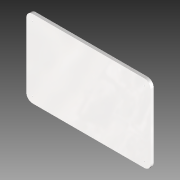
# Autodesk Inventor part: 4103_Aluminum Box Bottom_V1
Saved by Autodesk Inventor 2020 (Build 240168000, 168)
## iProperties
Created: 2020-09-13
Part Number: 4103_Aluminum Box Bottom_V1
Material: UHMW, White
Document SubType Name: Modeling
Designer: Eli Mattingly
Density: 0.94 g/cm^3
Appearance: Smooth - White
Author: Eli Mattingly
Autodesk Inventor part; units mm, degrees
ref_plane "YZ Plane" through (0, 0, 0) normal (1, 0, 0) x (0, 1, 0)
ref_plane "XZ Plane" through (0, 0, 0) normal (0, 1, 0) x (-1, 0, 0)
ref_plane "XY Plane" through (0, 0, 0) normal (0, 0, 1) x (1, 0, 0)
sketch "Sketch1" plane through (0, 0, 0) normal (0, 0, 1) x (1, 0, 0)
  line L0 (-200, 125) -> (200, 125)
  line L1 (200, 125) -> (200, -125)
  line L2 (200, -125) -> (-200, -125)
  line L3 (-200, -125) -> (-200, 125)
  line L4 (-200, 125) -> (200, -125) construction
  line L5 (200, 125) -> (-200, -125) construction
  point P0 (0, 0)
  dimension "d0" = 400
  dimension "d1" = 250
  constraints: 12 end point, 2 midpoint, 2 parallel, 1 horizontal, 1 perpendicular
  measures "d0" distance of L1.end L2.end
  measures "d1" distance of L0.end L1.end
extrude "Extrusion1" add sketch "Sketch1" against normal mid plane 10
fillet "Fillet1" radius 20 4 edges at (-200, -125, 0) (200, -125, 0) (200, 125, 0) (-200, 125, 0)
sketch "Sketch2" plane through (0, 0, 5) normal (0, 0, 1) x (1, 0, 0)
  arc A0 (-180, 125) -> (-200, 105) centre (-180, 105) ccw projected
  arc A1 (-200, -105) -> (-180, -125) centre (-180, -105) ccw projected
  arc A2 (180, -125) -> (200, -105) centre (180, -105) ccw projected
  arc A3 (200, 105) -> (180, 125) centre (180, 105) ccw projected
  point P0 (0, 0)
  constraints: 4 coincident
hole "Hole1" at (-180, 105, 5) at (180, 105, 5) at (180, -105, 5) at (-180, -105, 5) direction (0, 0, -1) diameter 4 end through all
body "Solid1"
